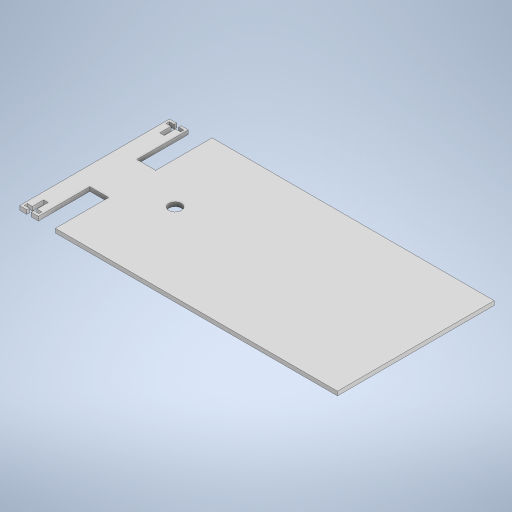
# Autodesk Inventor part: suelo_imp
Saved by Autodesk Inventor 2024 (Build 280153000, 153)
## iProperties
Created: 2023-05-01
Part Number: suelo_imp
Material: Generic
Document SubType Name: Modeling
Designer: Diego
Density: 1 g/cm^3
Appearance: Default
Author: Diego
Autodesk Inventor part; units mm, degrees
ref_plane "YZ Plane" through (0, 0, 0) normal (1, 0, 0) x (0, 1, 0)
ref_plane "XZ Plane" through (0, 0, 0) normal (0, 1, 0) x (-1, 0, 0)
ref_plane "XY Plane" through (0, 0, 0) normal (0, 0, 1) x (1, 0, 0)
sketch "Sketch1" plane through (0, 0, 0) normal (0, 1, 0) x (-1, 0, 0)
  line L0 (-97.5, -62.5) -> (97.5, -62.5)
  line L1 (97.5, 62.5) -> (-97.5, 62.5)
  line L2 (-97.5, 62.5) -> (-97.5, -62.5)
  line L3 (-97.5, -62.5) -> (97.5, 62.5) construction
  line L4 (97.5, -62.5) -> (-97.5, 62.5) construction
  line L5 (97.5, 20) -> (112.525, 20)
  line L6 (127.475, 21.2237) -> (127.475, -18.7763)
  line L7 (112.525, -17.5526) -> (97.5, -17.5526)
  line L8 (97.5, -62.5) -> (97.5, -17.5526)
  line L9 (97.5, 20) -> (97.5, 62.5)
  line L10 (112.525, 20) -> (112.525, 61)
  line L11 (127.475, 61) -> (127.475, 21.2237)
  line L12 (127.475, 1.2237) -> (97.475, 1.2237) construction
  line L13 (112.525, -17.5526) -> (112.525, -58.5526)
  line L14 (127.475, -58.5526) -> (127.475, -18.7763)
  line L15 (119.975, 61) -> (121.775, 61) construction
  line L16 (121.775, 61) -> (121.775, 59)
  line L17 (118.225, 61) -> (118.225, 59)
  line L18 (121.775, 59) -> (125.775, 59)
  line L19 (125.775, 59) -> (125.775, 56.5)
  line L20 (125.775, 56.5) -> (121.775, 56.5)
  line L21 (121.775, 61) -> (121.775, 53) construction
  line L22 (119.975, 61) -> (119.975, 52.3078) construction
  line L23 (118.225, 59) -> (114.175, 59)
  line L24 (114.175, 59) -> (114.175, 56.5)
  line L25 (114.175, 56.5) -> (118.175, 56.5)
  line L26 (118.175, 56.5) -> (118.175, 53.5)
  line L27 (112.525, 61) -> (118.225, 61)
  line L28 (127.475, 61) -> (121.775, 61)
  line L29 (119.975, -58.5526) -> (121.775, -58.5526) construction
  line L30 (112.525, -58.5526) -> (118.225, -58.5526)
  line L31 (127.475, -58.5526) -> (121.775, -58.5526)
  line L32 (121.775, 56.5) -> (121.775, 47.5)
  line L33 (118.175, 53.5) -> (118.175, 47.5)
  line L34 (118.175, 47.5) -> (121.775, 47.5)
  line L35 (119.975, -58.5526) -> (121.775, -58.5526) construction
  line L36 (121.775, -58.5526) -> (121.775, -56.5526)
  line L37 (118.225, -58.5526) -> (118.225, -56.5526)
  line L38 (121.775, -56.5526) -> (125.775, -56.5526)
  line L39 (125.775, -56.5526) -> (125.775, -54.0526)
  line L40 (125.775, -54.0526) -> (121.775, -54.0526)
  line L41 (121.775, -58.5526) -> (121.775, -50.5526) construction
  line L42 (119.975, -58.5526) -> (119.975, -49.8604) construction
  line L43 (114.175, -54.0526) -> (118.175, -54.0526)
  line L44 (114.175, -56.5526) -> (114.175, -54.0526)
  line L45 (118.225, -56.5526) -> (114.175, -56.5526)
  line L46 (118.175, -54.0526) -> (118.175, -51.0526)
  line L47 (112.525, -58.5526) -> (118.225, -58.5526)
  line L48 (127.475, -58.5526) -> (121.775, -58.5526)
  line L49 (121.775, -54.0526) -> (121.775, -45.0526)
  line L50 (118.175, -51.0526) -> (118.175, -45.0526)
  line L51 (118.175, -45.0526) -> (121.775, -45.0526)
  line L52 (127.475, 61) -> (127.475, 79) construction
  line L53 (-97.5, 0) -> (-67.5, 0) construction
  line L54 (-67.5, 62.5) -> (-67.5, -62.5) construction
  line L55 (127.475, 79) -> (-67.5, 0) construction
  line L56 (127.475, -58.5526) -> (127.475, -76.5526) construction
  line L57 (127.475, -76.5526) -> (-67.5, 0) construction
  line L58 (-97.5, 62.5) -> (-117.5, 62.5)
  line L59 (-117.5, 62.5) -> (-117.5, -62.5)
  line L60 (-117.5, -62.5) -> (-97.5, -62.5)
  line L61 (-97.5, -62.5) -> (-97.5, 62.5)
  point P0 (0, 0)
  point P1 (121.775, 53.5)
  point P2 (121.775, -51.0526)
  point P3 (-97.5, -62.5)
  dimension "d0" = 195
  dimension "d1" = 125
  dimension "d3" = 30
  dimension "d4" = 40
  dimension "d5" = 15
  dimension "d6" = 41
  dimension "d11" = 7.5
  dimension "d12" = 1.8
  dimension "d13" = 1.75
  dimension "d14" = 2
  dimension "d15" = 2
  dimension "d17" = 2.5
  dimension "d18" = 8
  dimension "d19" = 3
  dimension "d21" = 30
  dimension "d22" = 8.6922
  dimension "d23" = 1.5
  dimension "d25" = 4
  dimension "d26" = 13.25
  dimension "d27" = 9
  dimension "d28" = 18
  dimension "d29" = 30
  dimension "d30" = 18
  dimension "d35" = 20
  dimension "d36" = 125
  constraints: 124 end point, 24 symmetric about line, 13 perpendicular, 7 horizontal, 6 parallel, 6 point on line, 5 vertical, 4 midpoint
  measures "d0" distance of L1.end L1.start
  measures "d1" distance of L1.start L0.end
  measures "d3" distance of L5.start L6.start
  measures "d4" distance of L6.start L6.end
  measures "d5" distance of L5.end L6.start
  measures "d6" distance of L5.end L10.end
  measures "d11" distance of L11.start L15.start
  measures "d12" distance of L15.end L15.start
  measures "d13" distance of L15.start L17.start
  measures "d14" distance of L15.end L16.end
  measures "d15" distance of L17.start L17.end
  measures "d17" distance of L18.end L19.end
  measures "d18" distance of L15.end L21.end
  measures "d19" distance of L20.end point (121.775, 53.5)
  measures "d21" distance from line of L12.end L11
  measures "d22" distance from line of L22.end L28
  measures "d23" distance between parallel lines of L28 L1
  measures "d25" distance of L16.end L18.end
  measures "d26" distance from line of L10.end L19
  measures "d27" distance of L20.end L32.end
  measures "d28" distance of L11.start L52.end
  measures "d29" distance of L53.start L53.end
  measures "d30" distance of L14.start L56.end
  measures "d35" distance of L60.end L59.end
  measures "d36" distance of L59.end L58.end
extrude "Extrusion1" add sketch "Sketch1" along normal blind 3.25 contours L2 L1 L9 L5 L10 L27 L17 L23 L24 L25 L26 L33 L34 L32 L20 L19 L18 L16 L28 L11 L6 L14 L31 L36 L38 L39 L40 L49 L51 L50 L46 L43 L44 L45 L37 L30 L13 L7 L8 L0
sketch "Sketch2" plane through (0, 3.25, 0) normal (0, 1, 0) x (1, 0, 0)
  line L0 (-127.475, 58.5526) -> (-127.475, -61) construction
  line L1 (-127.475, 0) -> (-64.475, 0) construction
  circle A0 centre (-64.475, 0) radius 5
  point P0 (0, 0)
  dimension "d31" = 63
  dimension "d32" = 10
  constraints: 2 end point, 1 centre point, 1 coincident, 1 perpendicular, 1 point on line
  measures "d31" distance of L1.start L1.end
  measures "d32" diameter of A0
extrude "Extrusion2" cut sketch "Sketch2" against normal blind 10
sketch "Sketch3" plane through (97.5, 0, 62.5) normal (1, 0, 0) x (0, 0, -1)
  line L0 (125, 0) -> (80.0526, 0) projected
  line L1 (0, 3.25) -> (125, 3.25)
  line L2 (125, 3.25) -> (125, 0)
  line L3 (125, 0) -> (0, 0)
  line L4 (0, 0) -> (0, 3.25)
  point P0 (62.5, 0)
  constraints: 8 end point, 2 parallel, 1 horizontal, 1 perpendicular
extrude "Extrusion4" add sketch "Sketch3" along normal blind 30
body "Solid1"
